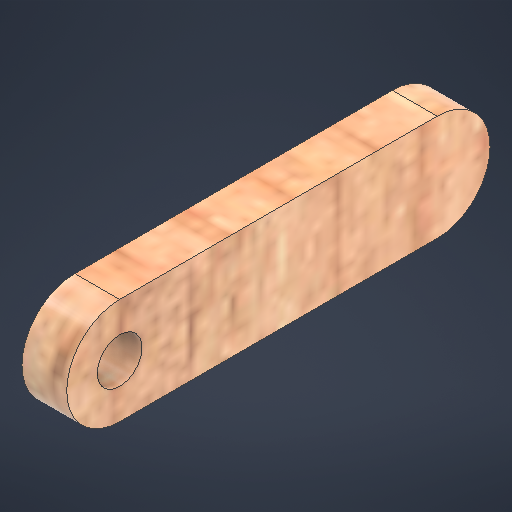
# Autodesk Inventor part: Lower Leg Skiba
Saved by Autodesk Inventor 2026.2 (Build 302298000, 298)
## iProperties
Created: 2024-10-30
Part Number: Lower Leg Skiba
Material: Generic
Document SubType Name: Modeling
Designer: 239tr
Density: 1 g/cm^3
Appearance: Birch - Natural Polished
Author: 239tr
Autodesk Inventor part; units mm, degrees
ref_plane "YZ Plane" through (0, 0, 0) normal (1, 0, 0) x (0, 1, 0)
ref_plane "XZ Plane" through (0, 0, 0) normal (0, 1, 0) x (-1, 0, 0)
ref_plane "XY Plane" through (0, 0, 0) normal (0, 0, 1) x (1, 0, 0)
sketch "Sketch1" plane through (0, 0, 0) normal (1, 0, 0) x (0, 1, 0)
  circle A0 centre (0, 0) radius 3.175
  arc A1 (7.5, 0) -> (-7.5, 0) centre (0, 0) ccw
  line L0 (7.5, 0) -> (7.5, -45)
  line L1 (-7.5, 0) -> (-7.5, -45)
  arc A2 (-7.5, -45) -> (7.5, -45) centre (0, -45) ccw
  circle A3 centre (0, -45) radius 3.175
  dimension "d0" = 6.35
  dimension "d1" = 15
  dimension "d2" = 15
  dimension "d3" = 45
  dimension "d4" = 6.35
  constraints: 4 centre point, 4 end point, 4 point on circle, 3 coincident, 3 tangent, 2 vertical
  measures "d0" diameter of A0
  measures "d1" diameter of A1
  measures "d2" diameter of A2
  measures "d3" distance of A2.centre A1.centre
  measures "d4" diameter of A3
extrude "Extrusion1" add sketch "Sketch1" along normal blind 6.35 contours L0 A2 L1 A1 | A3
body "Solid1"
